Autodesk Fusion 360 part; units mm, degrees
(part 3 of 6)
sketch "Sketch23" plane through (0, 3, 0) normal (0, 1, 0) x (-1, 0, 0)
  line L0 (75.3451, 40.8932) -> (75.3451, 33.735)
  line L1 (75.3451, 33.735) -> (70.1693, 33.735)
  line L2 (70.1693, 33.735) -> (70.1693, 34.5798)
  line L3 (70.1693, 34.5798) -> (74.3978, 34.5798)
  line L4 (74.3978, 34.5798) -> (74.3978, 36.7721)
  line L5 (74.3978, 36.7721) -> (70.4379, 36.7721)
  line L6 (70.4379, 36.7721) -> (70.4379, 37.612)
  line L7 (70.4379, 37.612) -> (74.3978, 37.612)
  line L8 (74.3978, 37.612) -> (74.3978, 40.0485)
  line L9 (74.3978, 40.0485) -> (70.0033, 40.0485)
  line L10 (70.0033, 40.0485) -> (70.0033, 40.8932)
  line L11 (70.0033, 40.8932) -> (75.3451, 40.8932)
  line L12 (61.3265, 40.1071) -> (61.1996, 40.8835)
  spline S0 degree 3 poles (61.1996, 40.8835) (61.3164, 40.9062) (61.5358, 40.949) (61.7592, 40.9576) (61.8636, 40.9616) knots 0 0 0 0 0.035641 0.066952 0.066952 0.066952 0.066952
  spline S1 degree 3 poles (61.8636, 40.9616) (62.0074, 40.9588) (62.2648, 40.9539) (62.5014, 40.8542) (62.6058, 40.8102) knots 0 0 0 0 0.042649 0.076356 0.076356 0.076356 0.076356
  spline S2 degree 3 poles (62.6058, 40.8102) (62.6866, 40.7573) (62.8429, 40.6547) (62.9332, 40.4913) (62.9769, 40.4123) knots 0 0 0 0 0.028484 0.055146 0.055146 0.055146 0.055146
  spline S3 degree 3 poles (62.9769, 40.4123) (63.0078, 40.2852) (63.0904, 39.9452) (63.0867, 39.5944) (63.0843, 39.3747) knots 0 0 0 0 0.039108 0.104654 0.104654 0.104654 0.104654
  line L13 (63.0843, 39.3747) -> (63.0843, 36.3913)
  line L14 (63.0843, 36.3913) -> (63.7289, 36.3913)
  line L15 (63.7289, 36.3913) -> (63.7289, 35.7077)
  line L16 (63.7289, 35.7077) -> (63.0843, 35.7077)
  line L17 (63.0843, 35.7077) -> (63.0843, 34.4235)
  line L18 (63.0843, 34.4235) -> (62.2103, 33.8962)
  line L19 (62.2103, 33.8962) -> (62.2103, 35.7077)
  line L20 (62.2103, 35.7077) -> (61.3265, 35.7077)
  line L21 (61.3265, 35.7077) -> (61.3265, 36.3913)
  line L22 (61.3265, 36.3913) -> (62.2103, 36.3913)
  line L23 (62.2103, 36.3913) -> (62.2103, 39.4235)
  spline S4 degree 3 poles (62.2103, 39.4235) (62.2116, 39.5271) (62.2137, 39.6903) (62.1772, 39.8489) (62.1639, 39.9069) knots 0 0 0 0 0.030906 0.048705 0.048705 0.048705 0.048705
  spline S5 degree 3 poles (62.1639, 39.9069) (62.1458, 39.941) (62.1091, 40.0101) (62.045, 40.0551) (62.0126, 40.0778) knots 0 0 0 0 0.011413 0.023119 0.023119 0.023119 0.023119
  spline S6 degree 3 poles (62.0126, 40.0778) (61.9706, 40.0963) (61.8753, 40.1382) (61.7708, 40.1402) (61.7123, 40.1413) knots 0 0 0 0 0.013616 0.030961 0.030961 0.030961 0.030961
  spline S7 degree 3 poles (61.7123, 40.1413) (61.6556, 40.1393) (61.5265, 40.1347) (61.3984, 40.117) (61.3265, 40.1071) knots 0 0 0 0 0.016989 0.038747 0.038747 0.038747 0.038747
  line L24 (54.9154, 40.8932) -> (54.9154, 35.7077)
  line L25 (54.9154, 35.7077) -> (54.1244, 35.7077)
  line L26 (54.1244, 35.7077) -> (54.1244, 36.4938)
  spline S8 degree 3 poles (54.1244, 36.4938) (54.0363, 36.3341) (53.8864, 36.0624) (53.659, 35.8527) (53.5653, 35.7663) knots 0 0 0 0 0.05425 0.092273 0.092273 0.092273 0.092273
  spline S9 degree 3 poles (53.5653, 35.7663) (53.4779, 35.715) (53.3035, 35.6128) (53.1019, 35.5979) (53.0013, 35.5905) knots 0 0 0 0 0.029972 0.059777 0.059777 0.059777 0.059777
  spline S10 degree 3 poles (53.0013, 35.5905) (52.8491, 35.6045) (52.5282, 35.6341) (52.2462, 35.7912) (52.098, 35.8737) knots 0 0 0 0 0.045356 0.095599 0.095599 0.095599 0.095599
  line L27 (52.098, 35.8737) -> (52.4008, 36.6891)
  spline S11 degree 3 poles (52.4008, 36.6891) (52.5059, 36.6336) (52.7082, 36.5268) (52.9359, 36.5078) (53.0453, 36.4987) knots 0 0 0 0 0.03525 0.067826 0.067826 0.067826 0.067826
  spline S12 degree 3 poles (53.0453, 36.4987) (53.1389, 36.5059) (53.3259, 36.5203) (53.4839, 36.6215) (53.5629, 36.672) knots 0 0 0 0 0.027685 0.055345 0.055345 0.055345 0.055345
  spline S13 degree 3 poles (53.5629, 36.672) (53.6343, 36.7369) (53.7818, 36.8708) (53.8532, 37.057) (53.89, 37.153) knots 0 0 0 0 0.028537 0.058895 0.058895 0.058895 0.058895
  spline S14 degree 3 poles (53.89, 37.153) (53.9327, 37.3157) (54.021, 37.6518) (54.0312, 37.9992) (54.0365, 38.1784) knots 0 0 0 0 0.050287 0.103879 0.103879 0.103879 0.103879
  line L28 (54.0365, 38.1784) -> (54.0365, 40.8932)
  line L29 (54.0365, 40.8932) -> (54.9154, 40.8932)
  line L30 (31.9125, 39.2233) -> (31.0043, 39.3356)
  spline S15 degree 3 poles (31.0043, 39.3356) (31.0877, 39.5834) (31.2492, 40.0629) (31.6207, 40.4055) (31.8002, 40.571) knots 0 0 0 0 0.077034 0.149075 0.149075 0.149075 0.149075
  spline S16 degree 3 poles (31.8002, 40.571) (32.0151, 40.699) (32.4715, 40.9709) (33.0033, 40.9968) (33.2845, 41.0104) knots 0 0 0 0 0.073917 0.156923 0.156923 0.156923 0.156923
  spline S17 degree 3 poles (33.2845, 41.0104) (33.6385, 40.987) (34.3153, 40.9421) (34.8389, 40.514) (35.0887, 40.3097) knots 0 0 0 0 0.103483 0.197891 0.197891 0.197891 0.197891
  spline S18 degree 3 poles (35.0887, 40.3097) (35.2829, 40.039) (35.7022, 39.454) (35.7367, 38.7321) (35.7552, 38.3444) knots 0 0 0 0 0.097893 0.211487 0.211487 0.211487 0.211487
  spline S19 degree 3 poles (35.7552, 38.3444) (35.737, 37.9438) (35.703, 37.2003) (35.2776, 36.5932) (35.0814, 36.3132) knots 0 0 0 0 0.117426 0.217964 0.217964 0.217964 0.217964
  spline S20 degree 3 poles (35.0814, 36.3132) (34.8361, 36.1024) (34.3334, 35.6707) (33.6719, 35.6177) (33.3334, 35.5905) knots 0 0 0 0 0.094484 0.193557 0.193557 0.193557 0.193557
  spline S21 degree 3 poles (33.3334, 35.5905) (33.0049, 35.6175) (32.3613, 35.6704) (31.8732, 36.092) (31.6342, 36.2985) knots 0 0 0 0 0.096126 0.18838 0.18838 0.18838 0.18838
  spline S22 degree 3 poles (31.6342, 36.2985) (31.4422, 36.5731) (31.0258, 37.1688) (30.9928, 37.8977) (30.975, 38.2907) knots 0 0 0 0 0.098509 0.213708 0.213708 0.213708 0.213708
  spline S23 degree 3 poles (30.975, 38.2907) (30.9753, 38.3233) (30.976, 38.4014) (30.9784, 38.4795) (30.9799, 38.5251) knots 0 0 0 0 0.009766 0.023443 0.023443 0.023443 0.023443
  line L31 (30.9799, 38.5251) -> (34.847, 38.5251)
  spline S24 degree 3 poles (34.847, 38.5251) (34.8216, 38.7854) (34.7748, 39.2658) (34.4928, 39.6553) (34.3636, 39.8337) knots 0 0 0 0 0.076825 0.141746 0.141746 0.141746 0.141746
  spline S25 degree 3 poles (34.3636, 39.8337) (34.2089, 39.9661) (33.8964, 40.2335) (33.4865, 40.2696) (33.2797, 40.2878) knots 0 0 0 0 0.059532 0.120175 0.120175 0.120175 0.120175
  spline S26 degree 3 poles (33.2797, 40.2878) (33.1265, 40.2787) (32.8304, 40.2612) (32.5769, 40.1079) (32.4545, 40.0339) knots 0 0 0 0 0.045247 0.087501 0.087501 0.087501 0.087501
  spline S27 degree 3 poles (32.4545, 40.0339) (32.3441, 39.9297) (32.1023, 39.7015) (31.9793, 39.3917) (31.9125, 39.2233) knots 0 0 0 0 0.045001 0.098557 0.098557 0.098557 0.098557
  line L32 (39.3357, 58.6816) -> (39.3357, 47.9224)
  line L33 (39.3357, 47.9224) -> (38.1345, 47.9224)
  line L34 (38.1345, 47.9224) -> (38.1345, 48.9331)
  spline S28 degree 3 poles (38.1345, 48.9331) (37.9928, 48.7502) (37.7217, 48.4005) (37.3516, 48.1586) (37.1751, 48.0432) knots 0 0 0 0 0.068849 0.131677 0.131677 0.131677 0.131677
  spline S29 degree 3 poles (37.1751, 48.0432) (36.9808, 47.9568) (36.5687, 47.7734) (36.1173, 47.7558) (35.8787, 47.7466) knots 0 0 0 0 0.063189 0.134074 0.134074 0.134074 0.134074
  spline S30 degree 3 poles (35.8787, 47.7466) (35.5593, 47.766) (34.9341, 47.8041) (34.388, 48.1098) (34.1209, 48.2593) knots 0 0 0 0 0.094622 0.185218 0.185218 0.185218 0.185218
  spline S31 degree 3 poles (34.1209, 48.2593) (33.881, 48.4515) (33.3885, 48.8462) (33.1125, 49.4144) (32.971, 49.7058) knots 0 0 0 0 0.091026 0.186859 0.186859 0.186859 0.186859
  spline S32 degree 3 poles (32.971, 49.7058) (32.8578, 50.0289) (32.6256, 50.6916) (32.5973, 51.3934) (32.5828, 51.7529) knots 0 0 0 0 0.102108 0.20939 0.20939 0.20939 0.20939
  spline S33 degree 3 poles (32.5828, 51.7529) (32.5981, 52.1352) (32.6277, 52.8747) (32.8863, 53.5678) (33.0112, 53.9026) knots 0 0 0 0 0.113938 0.220434 0.220434 0.220434 0.220434
  spline S34 degree 3 poles (33.0112, 53.9026) (33.167, 54.2005) (33.4717, 54.7833) (33.9988, 55.1757) (34.2564, 55.3674) knots 0 0 0 0 0.099433 0.194467 0.194467 0.194467 0.194467
  spline S35 degree 3 poles (34.2564, 55.3674) (34.5294, 55.5159) (35.066, 55.8077) (35.6748, 55.8538) (35.9739, 55.8765) knots 0 0 0 0 0.09206 0.180958 0.180958 0.180958 0.180958
  spline S36 degree 3 poles (35.9739, 55.8765) (36.1854, 55.8662) (36.5971, 55.8462) (36.9737, 55.6793) (37.1567, 55.5981) knots 0 0 0 0 0.062916 0.122451 0.122451 0.122451 0.122451
  spline S37 degree 3 poles (37.1567, 55.5981) (37.3222, 55.501) (37.6455, 55.311) (37.8953, 55.0315) (38.0173, 54.895) knots 0 0 0 0 0.057158 0.111733 0.111733 0.111733 0.111733
  line L35 (38.0173, 54.895) -> (38.0173, 58.6816)
  line L36 (38.0173, 58.6816) -> (39.3357, 58.6816)
  line L37 (25.991, 46.4795) -> (25.991, 44.9634)
  line L38 (25.991, 44.9634) -> (24.6726, 44.9634)
  line L39 (24.6726, 44.9634) -> (24.6726, 46.4795)
  line L40 (24.6726, 46.4795) -> (25.991, 46.4795)
  line L41 (23.1931, 53.3789) -> (21.8894, 53.1738)
  spline S38 degree 3 poles (21.8894, 53.1738) (21.8413, 53.4156) (21.75, 53.8747) (21.4295, 54.2143) (21.2778, 54.375) knots 0 0 0 0 0.072267 0.137238 0.137238 0.137238 0.137238
  spline S39 degree 3 poles (21.2778, 54.375) (21.0827, 54.4965) (20.6552, 54.7628) (20.1499, 54.782) (19.8753, 54.7925) knots 0 0 0 0 0.067812 0.148597 0.148597 0.148597 0.148597
  spline S40 degree 3 poles (19.8753, 54.7925) (19.6043, 54.7862) (19.1216, 54.7751) (18.7087, 54.5301) (18.5276, 54.4226) knots 0 0 0 0 0.07964 0.141834 0.141834 0.141834 0.141834
  spline S41 degree 3 poles (18.5276, 54.4226) (18.3995, 54.2977) (18.1534, 54.0576) (18.1093, 53.7177) (18.0881, 53.5547) knots 0 0 0 0 0.051978 0.099855 0.099855 0.099855 0.099855
  spline S42 degree 3 poles (18.0881, 53.5547) (18.1051, 53.4132) (18.1394, 53.1267) (18.3631, 52.944) (18.4763, 52.8516) knots 0 0 0 0 0.04108 0.083169 0.083169 0.083169 0.083169
  spline S43 degree 3 poles (18.4763, 52.8516) (18.6325, 52.7814) (19.0657, 52.5869) (19.5282, 52.4758) (19.824, 52.4048) knots 0 0 0 0 0.051284 0.142232 0.142232 0.142232 0.142232
  spline S44 degree 3 poles (19.824, 52.4048) (20.2366, 52.3014) (20.9198, 52.1303) (21.575, 51.8731) (21.8345, 51.7712) knots 0 0 0 0 0.127433 0.210981 0.210981 0.210981 0.210981
  spline S45 degree 3 poles (21.8345, 51.7712) (22.0084, 51.6761) (22.346, 51.4914) (22.5737, 51.1817) (22.6841, 51.0315) knots 0 0 0 0 0.058662 0.113875 0.113875 0.113875 0.113875
  spline S46 degree 3 poles (22.6841, 51.0315) (22.7685, 50.8691) (22.9386, 50.5418) (22.9617, 50.1734) (22.9734, 49.9878) knots 0 0 0 0 0.054242 0.109375 0.109375 0.109375 0.109375
  spline S47 degree 3 poles (22.9734, 49.9878) (22.9638, 49.8183) (22.9449, 49.4823) (22.8048, 49.1763) (22.7354, 49.0247) knots 0 0 0 0 0.050432 0.099993 0.099993 0.099993 0.099993
  spline S48 degree 3 poles (22.7354, 49.0247) (22.6488, 48.8832) (22.4756, 48.6001) (22.2167, 48.3924) (22.0872, 48.2886) knots 0 0 0 0 0.049345 0.098743 0.098743 0.098743 0.098743
  spline S49 degree 3 poles (22.0872, 48.2886) (21.9683, 48.2138) (21.706, 48.0488) (21.4103, 47.9552) (21.2485, 47.904) knots 0 0 0 0 0.04196 0.092591 0.092591 0.092591 0.092591
  spline S50 degree 3 poles (21.2485, 47.904) (21.0661, 47.8581) (20.6922, 47.7641) (20.3069, 47.7525) (20.1096, 47.7466) knots 0 0 0 0 0.056276 0.115276 0.115276 0.115276 0.115276
  spline S51 degree 3 poles (20.1096, 47.7466) (19.8208, 47.755) (19.2727, 47.7709) (18.7494, 47.9334) (18.502, 48.0103) knots 0 0 0 0 0.08622 0.163589 0.163589 0.163589 0.163589
  spline S52 degree 3 poles (18.502, 48.0103) (18.2913, 48.0995) (17.8993, 48.2656) (17.6128, 48.5793) (17.4802, 48.7244) knots 0 0 0 0 0.067685 0.125961 0.125961 0.125961 0.125961
  spline S53 degree 3 poles (17.4802, 48.7244) (17.3776, 48.896) (17.1541, 49.2697) (17.0711, 49.6978) (17.0261, 49.9292) knots 0 0 0 0 0.059547 0.129628 0.129628 0.129628 0.129628
  line L42 (17.0261, 49.9292) -> (18.3152, 50.105)
  spline S54 degree 3 poles (18.3152, 50.105) (18.3559, 49.9178) (18.4349, 49.5552) (18.6973, 49.2939) (18.8242, 49.1675) knots 0 0 0 0 0.056141 0.108715 0.108715 0.108715 0.108715
  spline S55 degree 3 poles (18.8242, 49.1675) (18.9894, 49.0694) (19.3548, 48.8527) (19.781, 48.8384) (20.0144, 48.8306) knots 0 0 0 0 0.056748 0.125473 0.125473 0.125473 0.125473
  spline S56 degree 3 poles (20.0144, 48.8306) (20.2797, 48.8327) (20.7368, 48.8364) (21.1412, 49.0438) (21.3108, 49.1309) knots 0 0 0 0 0.078181 0.134683 0.134683 0.134683 0.134683
  spline S57 degree 3 poles (21.3108, 49.1309) (21.4239, 49.2309) (21.6378, 49.4202) (21.6794, 49.7014) (21.699, 49.834) knots 0 0 0 0 0.043702 0.082651 0.082651 0.082651 0.082651
  spline S58 degree 3 poles (21.699, 49.834) (21.6921, 49.9175) (21.6784, 50.0852) (21.5848, 50.2251) (21.5379, 50.2954) knots 0 0 0 0 0.024684 0.0496 0.0496 0.0496 0.0496
  spline S59 degree 3 poles (21.5379, 50.2954) (21.4722, 50.3648) (21.3286, 50.5167) (21.1367, 50.6011) (21.0325, 50.647) knots 0 0 0 0 0.02837 0.062115 0.062115 0.062115 0.062115
  spline S60 degree 3 poles (21.0325, 50.647) (20.9027, 50.6879) (20.5172, 50.8093) (20.1268, 50.9143) (19.8679, 50.9839) knots 0 0 0 0 0.040831 0.121242 0.121242 0.121242 0.121242
  spline S61 degree 3 poles (19.8679, 50.9839) (19.4697, 51.0896) (18.8099, 51.2649) (18.1698, 51.5016) (17.916, 51.5955) knots 0 0 0 0 0.123506 0.204645 0.204645 0.204645 0.204645
  spline S62 degree 3 poles (17.916, 51.5955) (17.7429, 51.682) (17.4043, 51.8513) (17.165, 52.1444) (17.0481, 52.2876) knots 0 0 0 0 0.057342 0.11214 0.11214 0.11214 0.11214
  spline S63 degree 3 poles (17.0481, 52.2876) (16.9563, 52.4535) (16.7625, 52.8039) (16.7433, 53.2046) (16.7332, 53.4155) knots 0 0 0 0 0.056117 0.118505 0.118505 0.118505 0.118505
  spline S64 degree 3 poles (16.7332, 53.4155) (16.7501, 53.6335) (16.7846, 54.0761) (17.0055, 54.4614) (17.1177, 54.657) knots 0 0 0 0 0.064713 0.13142 0.13142 0.13142 0.13142
  spline S65 degree 3 poles (17.1177, 54.657) (17.2639, 54.8417) (17.5664, 55.2241) (18.0021, 55.4441) (18.2273, 55.5579) knots 0 0 0 0 0.0698 0.14446 0.14446 0.14446 0.14446
  spline S66 degree 3 poles (18.2273, 55.5579) (18.4822, 55.6507) (19.0119, 55.8437) (19.5756, 55.8653) (19.8679, 55.8765) knots 0 0 0 0 0.080881 0.168038 0.168038 0.168038 0.168038
  spline S67 degree 3 poles (19.8679, 55.8765) (20.3248, 55.8636) (21.1496, 55.8403) (21.8612, 55.4297) (22.1787, 55.2466) knots 0 0 0 0 0.1345 0.242846 0.242846 0.242846 0.242846
  spline S68 degree 3 poles (22.1787, 55.2466) (22.4214, 55.0003) (22.9373, 54.4768) (23.1046, 53.759) (23.1931, 53.3789) knots 0 0 0 0 0.101736 0.21624 0.21624 0.21624 0.21624
  line L43 (25.991, 55.7007) -> (25.991, 47.9224)
  line L44 (25.991, 47.9224) -> (24.6726, 47.9224)
  line L45 (24.6726, 47.9224) -> (24.6726, 55.7007)
  line L46 (24.6726, 55.7007) -> (25.991, 55.7007)
  line L47 (31.0081, 55.7007) -> (31.0081, 47.9224)
  line L48 (31.0081, 47.9224) -> (29.8215, 47.9224)
  line L49 (29.8215, 47.9224) -> (29.8215, 49.1016)
  spline S69 degree 3 poles (29.8215, 49.1016) (29.6894, 48.862) (29.4646, 48.4545) (29.1235, 48.1399) (28.9829, 48.0103) knots 0 0 0 0 0.081375 0.138409 0.138409 0.138409 0.138409
  spline S70 degree 3 poles (28.9829, 48.0103) (28.8518, 47.9333) (28.5902, 47.78) (28.2878, 47.7577) (28.137, 47.7466) knots 0 0 0 0 0.044958 0.089666 0.089666 0.089666 0.089666
  spline S71 degree 3 poles (28.137, 47.7466) (27.9086, 47.7676) (27.4272, 47.812) (27.0043, 48.0476) (26.782, 48.1714) knots 0 0 0 0 0.068034 0.143398 0.143398 0.143398 0.143398
  line L50 (26.782, 48.1714) -> (27.2361, 49.3945)
  spline S72 degree 3 poles (27.2361, 49.3945) (27.3938, 49.3113) (27.6972, 49.151) (28.0388, 49.1226) (28.2029, 49.1089) knots 0 0 0 0 0.052874 0.101739 0.101739 0.101739 0.101739
  spline S73 degree 3 poles (28.2029, 49.1089) (28.3432, 49.1197) (28.6238, 49.1413) (28.8608, 49.2931) (28.9793, 49.3689) knots 0 0 0 0 0.041528 0.083017 0.083017 0.083017 0.083017
  spline S74 degree 3 poles (28.9793, 49.3689) (29.0865, 49.4662) (29.3077, 49.667) (29.4148, 49.9464) (29.47, 50.0903) knots 0 0 0 0 0.042806 0.088343 0.088343 0.088343 0.088343
  spline S75 degree 3 poles (29.47, 50.0903) (29.534, 50.3344) (29.6664, 50.8385) (29.6818, 51.3596) (29.6897, 51.6284) knots 0 0 0 0 0.075431 0.155819 0.155819 0.155819 0.155819
  line L51 (29.6897, 51.6284) -> (29.6897, 55.7007)
  line L52 (29.6897, 55.7007) -> (31.0081, 55.7007)
  line L53 (47.3484, 53.1958) -> (45.9861, 53.3643)
  spline S76 degree 3 poles (45.9861, 53.3643) (46.1113, 53.7359) (46.3535, 54.4552) (46.9107, 54.969) (47.1799, 55.2173) knots 0 0 0 0 0.115551 0.223613 0.223613 0.223613 0.223613
  spline S77 degree 3 poles (47.1799, 55.2173) (47.5024, 55.4094) (48.1869, 55.8172) (48.9846, 55.8559) (49.4065, 55.8765) knots 0 0 0 0 0.110875 0.235384 0.235384 0.235384 0.235384
  spline S78 degree 3 poles (49.4065, 55.8765) (49.9374, 55.8413) (50.9526, 55.774) (51.7381, 55.1318) (52.1128, 54.8254) knots 0 0 0 0 0.155225 0.296837 0.296837 0.296837 0.296837
  spline S79 degree 3 poles (52.1128, 54.8254) (52.404, 54.4193) (53.033, 53.5417) (53.0848, 52.459) (53.1126, 51.8774) knots 0 0 0 0 0.146839 0.31723 0.31723 0.31723 0.31723
  spline S80 degree 3 poles (53.1126, 51.8774) (53.0851, 51.2766) (53.0342, 50.1613) (52.3961, 49.2506) (52.1018, 48.8306) knots 0 0 0 0 0.176138 0.326947 0.326947 0.326947 0.326947
  spline S81 degree 3 poles (52.1018, 48.8306) (51.7338, 48.5145) (50.9798, 47.8669) (49.9876, 47.7873) (49.4797, 47.7466) knots 0 0 0 0 0.141726 0.290335 0.290335 0.290335 0.290335
  spline S82 degree 3 poles (49.4797, 47.7466) (48.9871, 47.7871) (48.0216, 47.8664) (47.2895, 48.4989) (46.9309, 48.8086) knots 0 0 0 0 0.144189 0.28257 0.28257 0.28257 0.28257
  spline S83 degree 3 poles (46.9309, 48.8086) (46.643, 49.2205) (46.0184, 50.114) (45.9688, 51.2074) (45.9421, 51.7969) knots 0 0 0 0 0.147764 0.320562 0.320562 0.320562 0.320562
  spline S84 degree 3 poles (45.9421, 51.7969) (45.9426, 51.8457) (45.9437, 51.9629) (45.9474, 52.0801) (45.9495, 52.1484) knots 0 0 0 0 0.01465 0.035165 0.035165 0.035165 0.035165
  line L54 (45.9495, 52.1484) -> (51.7503, 52.1484)
  spline S85 degree 3 poles (51.7503, 52.1484) (51.7122, 52.539) (51.6419, 53.2596) (51.2189, 53.8438) (51.0252, 54.1113) knots 0 0 0 0 0.115238 0.212619 0.212619 0.212619 0.212619
  spline S86 degree 3 poles (51.0252, 54.1113) (50.793, 54.31) (50.3243, 54.711) (49.7094, 54.7652) (49.3992, 54.7925) knots 0 0 0 0 0.089299 0.180262 0.180262 0.180262 0.180262
  spline S87 degree 3 poles (49.3992, 54.7925) (49.1695, 54.7789) (48.7253, 54.7526) (48.345, 54.5227) (48.1614, 54.4116) knots 0 0 0 0 0.067871 0.131252 0.131252 0.131252 0.131252
  spline S88 degree 3 poles (48.1614, 54.4116) (47.9958, 54.2553) (47.6332, 53.913) (47.4487, 53.4483) (47.3484, 53.1958) knots 0 0 0 0 0.067501 0.147835 0.147835 0.147835 0.147835
  line L55 (65.1829, 55.7007) -> (65.1829, 47.9224)
  line L56 (65.1829, 47.9224) -> (63.9963, 47.9224)
  line L57 (63.9963, 47.9224) -> (63.9963, 49.0283)
  spline S89 degree 3 poles (63.9963, 49.0283) (63.6751, 48.6545) (63.0232, 47.8958) (62.0264, 47.7968) (61.5208, 47.7466) knots 0 0 0 0 0.142165 0.288537 0.288537 0.288537 0.288537
  spline S90 degree 3 poles (61.5208, 47.7466) (61.2936, 47.7561) (60.8496, 47.7746) (60.4319, 47.9256) (60.228, 47.9993) knots 0 0 0 0 0.067769 0.132408 0.132408 0.132408 0.132408
  spline S91 degree 3 poles (60.228, 47.9993) (60.0475, 48.0852) (59.7079, 48.2468) (59.4611, 48.5296) (59.3455, 48.6621) knots 0 0 0 0 0.059243 0.111422 0.111422 0.111422 0.111422
  spline S92 degree 3 poles (59.3455, 48.6621) (59.2545, 48.8083) (59.0662, 49.111) (58.9799, 49.4572) (58.9353, 49.6362) knots 0 0 0 0 0.051309 0.106275 0.106275 0.106275 0.106275
  spline S93 degree 3 poles (58.9353, 49.6362) (58.9142, 49.8039) (58.8606, 50.2292) (58.8615, 50.6581) (58.8621, 50.918) knots 0 0 0 0 0.050653 0.128494 0.128494 0.128494 0.128494
  line L58 (58.8621, 50.918) -> (58.8621, 55.7007)
  line L59 (58.8621, 55.7007) -> (60.1804, 55.7007)
  line L60 (60.1804, 55.7007) -> (60.1804, 50.9692)
  spline S94 degree 3 poles (60.1804, 50.9692) (60.1817, 50.7329) (60.1839, 50.3244) (60.2896, 49.9305) (60.3342, 49.7644) knots 0 0 0 0 0.070509 0.1219 0.1219 0.1219 0.1219
  spline S95 degree 3 poles (60.3342, 49.7644) (60.3966, 49.6373) (60.5238, 49.3784) (60.7597, 49.212) (60.8799, 49.1272) knots 0 0 0 0 0.04175 0.085098 0.085098 0.085098 0.085098
  spline S96 degree 3 poles (60.8799, 49.1272) (61.0192, 49.0578) (61.3084, 48.9137) (61.6316, 48.8975) (61.7991, 48.8892) knots 0 0 0 0 0.046164 0.095868 0.095868 0.095868 0.095868
  spline S97 degree 3 poles (61.7991, 48.8892) (62.0692, 48.9105) (62.6041, 48.9529) (63.0381, 49.2679) (63.2529, 49.4238) knots 0 0 0 0 0.079591 0.15761 0.15761 0.15761 0.15761
  spline S98 degree 3 poles (63.2529, 49.4238) (63.4301, 49.6738) (63.8559, 50.2745) (63.8613, 51.0183) (63.8645, 51.4526) knots 0 0 0 0 0.090016 0.216372 0.216372 0.216372 0.216372
  line L61 (63.8645, 51.4526) -> (63.8645, 55.7007)
  line L62 (63.8645, 55.7007) -> (65.1829, 55.7007)
  line L63 (77.2473, 74.5713) -> (77.2473, 60.2549)
  line L64 (77.2473, 60.2549) -> (66.8957, 60.2549)
  line L65 (66.8957, 60.2549) -> (66.8957, 61.9443)
  line L66 (66.8957, 61.9443) -> (75.3528, 61.9443)
  line L67 (75.3528, 61.9443) -> (75.3528, 66.3291)
  line L68 (75.3528, 66.3291) -> (67.4328, 66.3291)
  line L69 (67.4328, 66.3291) -> (67.4328, 68.0088)
  line L70 (67.4328, 68.0088) -> (75.3528, 68.0088)
  line L71 (75.3528, 68.0088) -> (75.3528, 72.8818)
  line L72 (75.3528, 72.8818) -> (66.5637, 72.8818)
  line L73 (66.5637, 72.8818) -> (66.5637, 74.5713)
  line L74 (66.5637, 74.5713) -> (77.2473, 74.5713)
  line L75 (49.2102, 72.999) -> (48.9563, 74.5517)
  spline S99 degree 3 poles (48.9563, 74.5517) (49.1899, 74.5972) (49.6288, 74.6827) (50.0755, 74.6999) (50.2844, 74.708) knots 0 0 0 0 0.071282 0.133904 0.133904 0.133904 0.133904
  spline S100 degree 3 poles (50.2844, 74.708) (50.5719, 74.7024) (51.0867, 74.6925) (51.5599, 74.4932) (51.7688, 74.4052) knots 0 0 0 0 0.085297 0.152712 0.152712 0.152712 0.152712
  spline S101 degree 3 poles (51.7688, 74.4052) (51.9303, 74.2993) (52.2429, 74.0941) (52.4236, 73.7673) (52.511, 73.6093) knots 0 0 0 0 0.056968 0.110293 0.110293 0.110293 0.110293
  spline S102 degree 3 poles (52.511, 73.6093) (52.5727, 73.3552) (52.738, 72.6752) (52.7305, 71.9736) (52.7258, 71.5341) knots 0 0 0 0 0.078216 0.209307 0.209307 0.209307 0.209307
  line L76 (52.7258, 71.5341) -> (52.7258, 65.5674)
  line L77 (52.7258, 65.5674) -> (54.0149, 65.5674)
  line L78 (54.0149, 65.5674) -> (54.0149, 64.2002)
  line L79 (54.0149, 64.2002) -> (52.7258, 64.2002)
  line L80 (52.7258, 64.2002) -> (52.7258, 61.6318)
  line L81 (52.7258, 61.6318) -> (50.9778, 60.5771)
  line L82 (50.9778, 60.5771) -> (50.9778, 64.2002)
  line L83 (50.9778, 64.2002) -> (49.2102, 64.2002)
  line L84 (49.2102, 64.2002) -> (49.2102, 65.5674)
  line L85 (49.2102, 65.5674) -> (50.9778, 65.5674)
  line L86 (50.9778, 65.5674) -> (50.9778, 71.6318)
  spline S103 degree 3 poles (50.9778, 71.6318) (50.9804, 71.8389) (50.9844, 72.1653) (50.9116, 72.4826) (50.885, 72.5986) knots 0 0 0 0 0.061811 0.09741 0.09741 0.09741 0.09741
  spline S104 degree 3 poles (50.885, 72.5986) (50.8488, 72.6668) (50.7753, 72.805) (50.6472, 72.8949) (50.5823, 72.9404) knots 0 0 0 0 0.022826 0.046239 0.046239 0.046239 0.046239
  spline S105 degree 3 poles (50.5823, 72.9404) (50.4984, 72.9773) (50.3077, 73.0612) (50.0987, 73.0651) (49.9817, 73.0674) knots 0 0 0 0 0.027232 0.061923 0.061923 0.061923 0.061923
  spline S106 degree 3 poles (49.9817, 73.0674) (49.8684, 73.0633) (49.6101, 73.0542) (49.354, 73.0188) (49.2102, 72.999) knots 0 0 0 0 0.033979 0.077495 0.077495 0.077495 0.077495
  line L87 (36.3879, 74.5713) -> (36.3879, 64.2002)
  line L88 (36.3879, 64.2002) -> (34.8059, 64.2002)
  line L89 (34.8059, 64.2002) -> (34.8059, 65.7724)
  spline S107 degree 3 poles (34.8059, 65.7724) (34.6297, 65.453) (34.3299, 64.9096) (33.8751, 64.4902) (33.6877, 64.3174) knots 0 0 0 0 0.1085 0.184546 0.184546 0.184546 0.184546
  spline S108 degree 3 poles (33.6877, 64.3174) (33.5128, 64.2148) (33.164, 64.0103) (32.7608, 63.9806) (32.5598, 63.9658) knots 0 0 0 0 0.059943 0.119555 0.119555 0.119555 0.119555
  spline S109 degree 3 poles (32.5598, 63.9658) (32.2553, 63.9939) (31.6135, 64.053) (31.0495, 64.3671) (30.7532, 64.5322) knots 0 0 0 0 0.090712 0.191197 0.191197 0.191197 0.191197
  line L90 (30.7532, 64.5322) -> (31.3586, 66.1631)
  spline S110 degree 3 poles (31.3586, 66.1631) (31.5689, 66.052) (31.9735, 65.8384) (32.4289, 65.8004) (32.6477, 65.7822) knots 0 0 0 0 0.070499 0.135652 0.135652 0.135652 0.135652
  spline S111 degree 3 poles (32.6477, 65.7822) (32.8348, 65.7966) (33.2089, 65.8254) (33.5249, 66.0278) (33.6828, 66.1289) knots 0 0 0 0 0.05537 0.110689 0.110689 0.110689 0.110689
  spline S112 degree 3 poles (33.6828, 66.1289) (33.8258, 66.2586) (34.1208, 66.5264) (34.2635, 66.8988) (34.3371, 67.0908) knots 0 0 0 0 0.057074 0.117791 0.117791 0.117791 0.117791
  spline S113 degree 3 poles (34.3371, 67.0908) (34.4226, 67.4162) (34.599, 68.0883) (34.6195, 68.7831) (34.6301, 69.1416) knots 0 0 0 0 0.100574 0.207758 0.207758 0.207758 0.207758
  line L91 (34.6301, 69.1416) -> (34.6301, 74.5713)
  line L92 (34.6301, 74.5713) -> (36.3879, 74.5713)
  line L93 (-9.6179, 71.2314) -> (-11.4343, 71.456)
  spline S114 degree 3 poles (-11.4343, 71.456) (-11.2675, 71.9516) (-10.9445, 72.9106) (-10.2016, 73.5957) (-9.8425, 73.9267) knots 0 0 0 0 0.154068 0.298151 0.298151 0.298151 0.298151
  spline S115 degree 3 poles (-9.8425, 73.9267) (-9.4126, 74.1828) (-8.4999, 74.7266) (-7.4364, 74.7783) (-6.8738, 74.8056) knots 0 0 0 0 0.147834 0.313845 0.313845 0.313845 0.313845
  spline S116 degree 3 poles (-6.8738, 74.8056) (-6.1659, 74.7587) (-4.8123, 74.669) (-3.765, 73.8128) (-3.2654, 73.4043) knots 0 0 0 0 0.206966 0.395783 0.395783 0.395783 0.395783
  spline S117 degree 3 poles (-3.2654, 73.4043) (-2.8772, 72.8627) (-2.0385, 71.6927) (-1.9695, 70.249) (-1.9324, 69.4736) knots 0 0 0 0 0.195785 0.422974 0.422974 0.422974 0.422974
  spline S118 degree 3 poles (-1.9324, 69.4736) (-1.9689, 68.6725) (-2.0368, 67.1854) (-2.8876, 65.9712) (-3.28, 65.4111) knots 0 0 0 0 0.234851 0.435929 0.435929 0.435929 0.435929
  spline S119 degree 3 poles (-3.28, 65.4111) (-3.7708, 64.9896) (-4.776, 64.1262) (-6.099, 64.0201) (-6.7761, 63.9658) knots 0 0 0 0 0.188967 0.387114 0.387114 0.387114 0.387114
  spline S120 degree 3 poles (-6.7761, 63.9658) (-7.433, 64.0198) (-8.7203, 64.1256) (-9.6965, 64.9688) (-10.1746, 65.3818) knots 0 0 0 0 0.192252 0.37676 0.37676 0.37676 0.37676
  spline S121 degree 3 poles (-10.1746, 65.3818) (-10.5585, 65.931) (-11.3913, 67.1223) (-11.4573, 68.5803) (-11.4929, 69.3662) knots 0 0 0 0 0.197018 0.427415 0.427415 0.427415 0.427415
  spline S122 degree 3 poles (-11.4929, 69.3662) (-11.4923, 69.4313) (-11.4908, 69.5876) (-11.486, 69.7438) (-11.4832, 69.8349) knots 0 0 0 0 0.019533 0.046886 0.046886 0.046886 0.046886
  line L94 (-11.4832, 69.8349) -> (-3.7488, 69.8349)
  spline S123 degree 3 poles (-3.7488, 69.8349) (-3.7996, 70.3557) (-3.8933, 71.3165) (-4.4573, 72.0954) (-4.7156, 72.4521) knots 0 0 0 0 0.153651 0.283492 0.283492 0.283492 0.283492
  spline S124 degree 3 poles (-4.7156, 72.4521) (-5.0252, 72.717) (-5.6501, 73.2517) (-6.4699, 73.3239) (-6.8836, 73.3603) knots 0 0 0 0 0.119065 0.24035 0.24035 0.24035 0.24035
  spline S125 degree 3 poles (-6.8836, 73.3603) (-7.1898, 73.3422) (-7.7821, 73.3072) (-8.2891, 73.0006) (-8.534, 72.8525) knots 0 0 0 0 0.090495 0.175003 0.175003 0.175003 0.175003
  spline S126 degree 3 poles (-8.534, 72.8525) (-8.7547, 72.6441) (-9.2382, 72.1877) (-9.4842, 71.5681) (-9.6179, 71.2314) knots 0 0 0 0 0.090002 0.197114 0.197114 0.197114 0.197114
  line L95 (80, 80) -> (-25, 80)
  line L96 (-25, 80) -> (-25, 30)
  line L97 (-25, 30) -> (80, 30)
  line L98 (80, 30) -> (80, 80)
  line L99 (64.1711, 74.5713) -> (64.1711, 64.2002)
  line L100 (64.1711, 64.2002) -> (62.5891, 64.2002)
  line L101 (62.5891, 64.2002) -> (62.5891, 65.6748)
  spline S127 degree 3 poles (62.5891, 65.6748) (62.1608, 65.1763) (61.2915, 64.1647) (59.9625, 64.0328) (59.2883, 63.9658) knots 0 0 0 0 0.189553 0.384716 0.384716 0.384716 0.384716
  spline S128 degree 3 poles (59.2883, 63.9658) (58.9854, 63.9785) (58.3935, 64.0032) (57.8366, 64.2045) (57.5647, 64.3027) knots 0 0 0 0 0.090359 0.176544 0.176544 0.176544 0.176544
  spline S129 degree 3 poles (57.5647, 64.3027) (57.3239, 64.4173) (56.8712, 64.6327) (56.5421, 65.0099) (56.3879, 65.1865) knots 0 0 0 0 0.078991 0.148563 0.148563 0.148563 0.148563
  spline S130 degree 3 poles (56.3879, 65.1865) (56.2667, 65.3814) (56.0155, 65.785) (55.9005, 66.2466) (55.841, 66.4853) knots 0 0 0 0 0.068412 0.1417 0.1417 0.1417 0.1417
  spline S131 degree 3 poles (55.841, 66.4853) (55.8129, 66.7089) (55.7414, 67.276) (55.7426, 67.8478) (55.7434, 68.1943) knots 0 0 0 0 0.067537 0.171325 0.171325 0.171325 0.171325
  line L102 (55.7434, 68.1943) -> (55.7434, 74.5713)
  line L103 (55.7434, 74.5713) -> (57.5012, 74.5713)
  line L104 (57.5012, 74.5713) -> (57.5012, 68.2627)
  spline S132 degree 3 poles (57.5012, 68.2627) (57.5029, 67.9476) (57.5058, 67.4028) (57.6468, 66.8776) (57.7063, 66.6562) knots 0 0 0 0 0.094012 0.162533 0.162533 0.162533 0.162533
  spline S133 degree 3 poles (57.7063, 66.6562) (57.7895, 66.4868) (57.959, 66.1415) (58.2736, 65.9196) (58.4338, 65.8066) knots 0 0 0 0 0.055666 0.113464 0.113464 0.113464 0.113464
  spline S134 degree 3 poles (58.4338, 65.8066) (58.6195, 65.7141) (59.0052, 65.5219) (59.436, 65.5004) (59.6594, 65.4892) knots 0 0 0 0 0.061552 0.127824 0.127824 0.127824 0.127824
  spline S135 degree 3 poles (59.6594, 65.4892) (60.0196, 65.5177) (60.7327, 65.5742) (61.3114, 65.9942) (61.5979, 66.2021) knots 0 0 0 0 0.106122 0.210147 0.210147 0.210147 0.210147
  spline S136 degree 3 poles (61.5979, 66.2021) (61.8341, 66.5354) (62.4018, 67.3364) (62.4091, 68.3281) (62.4133, 68.9072) knots 0 0 0 0 0.120022 0.288496 0.288496 0.288496 0.288496
  line L105 (62.4133, 68.9072) -> (62.4133, 74.5713)
  line L106 (62.4133, 74.5713) -> (64.1711, 74.5713)
  line L107 (40.3918, 71.2314) -> (38.5754, 71.456)
  spline S137 degree 3 poles (38.5754, 71.456) (38.7423, 71.9516) (39.0652, 72.9106) (39.8082, 73.5957) (40.1672, 73.9267) knots 0 0 0 0 0.154068 0.298151 0.298151 0.298151 0.298151
  spline S138 degree 3 poles (40.1672, 73.9267) (40.5971, 74.1828) (41.5099, 74.7266) (42.5734, 74.7783) (43.136, 74.8056) knots 0 0 0 0 0.147834 0.313845 0.313845 0.313845 0.313845
  spline S139 degree 3 poles (43.136, 74.8056) (43.8438, 74.7587) (45.1975, 74.669) (46.2447, 73.8128) (46.7444, 73.4043) knots 0 0 0 0 0.206966 0.395783 0.395783 0.395783 0.395783
  spline S140 degree 3 poles (46.7444, 73.4043) (47.1326, 72.8627) (47.9713, 71.6927) (48.0403, 70.249) (48.0774, 69.4736) knots 0 0 0 0 0.195785 0.422974 0.422974 0.422974 0.422974
  spline S141 degree 3 poles (48.0774, 69.4736) (48.0408, 68.6725) (47.973, 67.1854) (47.1222, 65.9712) (46.7297, 65.4111) knots 0 0 0 0 0.234851 0.435929 0.435929 0.435929 0.435929
  spline S142 degree 3 poles (46.7297, 65.4111) (46.239, 64.9896) (45.2337, 64.1262) (43.9108, 64.0201) (43.2336, 63.9658) knots 0 0 0 0 0.188967 0.387114 0.387114 0.387114 0.387114
  spline S143 degree 3 poles (43.2336, 63.9658) (42.5767, 64.0198) (41.2894, 64.1256) (40.3132, 64.9688) (39.8352, 65.3818) knots 0 0 0 0 0.192252 0.37676 0.37676 0.37676 0.37676
  spline S144 degree 3 poles (39.8352, 65.3818) (39.4513, 65.931) (38.6184, 67.1223) (38.5524, 68.5803) (38.5168, 69.3662) knots 0 0 0 0 0.197018 0.427415 0.427415 0.427415 0.427415
  spline S145 degree 3 poles (38.5168, 69.3662) (38.5175, 69.4313) (38.5189, 69.5876) (38.5238, 69.7438) (38.5266, 69.8349) knots 0 0 0 0 0.019533 0.046886 0.046886 0.046886 0.046886
  line L108 (38.5266, 69.8349) -> (46.261, 69.8349)
  spline S146 degree 3 poles (46.261, 69.8349) (46.2102, 70.3557) (46.1165, 71.3165) (45.5525, 72.0954) (45.2942, 72.4521) knots 0 0 0 0 0.153651 0.283492 0.283492 0.283492 0.283492
  spline S147 degree 3 poles (45.2942, 72.4521) (44.9846, 72.717) (44.3597, 73.2517) (43.5399, 73.3239) (43.1262, 73.3603) knots 0 0 0 0 0.119065 0.24035 0.24035 0.24035 0.24035
  spline S148 degree 3 poles (43.1262, 73.3603) (42.8199, 73.3422) (42.2277, 73.3072) (41.7207, 73.0006) (41.4758, 72.8525) knots 0 0 0 0 0.090495 0.175003 0.175003 0.175003 0.175003
  spline S149 degree 3 poles (41.4758, 72.8525) (41.255, 72.6441) (40.7715, 72.1877) (40.5255, 71.5681) (40.3918, 71.2314) knots 0 0 0 0 0.090002 0.197114 0.197114 0.197114 0.197114
  line L109 (18.6047, 74.5713) -> (18.6047, 64.2002)
  line L110 (18.6047, 64.2002) -> (17.0227, 64.2002)
  line L111 (17.0227, 64.2002) -> (17.0227, 65.7724)
  spline S150 degree 3 poles (17.0227, 65.7724) (16.8465, 65.453) (16.5467, 64.9096) (16.0919, 64.4902) (15.9045, 64.3174) knots 0 0 0 0 0.1085 0.184546 0.184546 0.184546 0.184546
  spline S151 degree 3 poles (15.9045, 64.3174) (15.7296, 64.2148) (15.3808, 64.0103) (14.9776, 63.9806) (14.7766, 63.9658) knots 0 0 0 0 0.059943 0.119555 0.119555 0.119555 0.119555
  spline S152 degree 3 poles (14.7766, 63.9658) (14.4721, 63.9939) (13.8303, 64.053) (13.2663, 64.3671) (12.97, 64.5322) knots 0 0 0 0 0.090712 0.191197 0.191197 0.191197 0.191197
  line L112 (12.97, 64.5322) -> (13.5754, 66.1631)
  spline S153 degree 3 poles (13.5754, 66.1631) (13.7857, 66.052) (14.1903, 65.8384) (14.6457, 65.8004) (14.8645, 65.7822) knots 0 0 0 0 0.070499 0.135652 0.135652 0.135652 0.135652
  spline S154 degree 3 poles (14.8645, 65.7822) (15.0516, 65.7966) (15.4257, 65.8254) (15.7417, 66.0278) (15.8996, 66.1289) knots 0 0 0 0 0.05537 0.110689 0.110689 0.110689 0.110689
  spline S155 degree 3 poles (15.8996, 66.1289) (16.0426, 66.2586) (16.3376, 66.5264) (16.4803, 66.8988) (16.5539, 67.0908) knots 0 0 0 0 0.057074 0.117791 0.117791 0.117791 0.117791
  spline S156 degree 3 poles (16.5539, 67.0908) (16.6394, 67.4162) (16.8158, 68.0883) (16.8363, 68.7831) (16.8469, 69.1416) knots 0 0 0 0 0.100574 0.207758 0.207758 0.207758 0.207758
  line L113 (16.8469, 69.1416) -> (16.8469, 74.5713)
  line L114 (16.8469, 74.5713) -> (18.6047, 74.5713)
  line L115 (11.9153, 74.5713) -> (11.9153, 64.2002)
  line L116 (11.9153, 64.2002) -> (10.1575, 64.2002)
  line L117 (10.1575, 64.2002) -> (10.1575, 74.5713)
  line L118 (10.1575, 74.5713) -> (11.9153, 74.5713)
  line L119 (8.1848, 71.4756) -> (6.4465, 71.2021)
  spline S157 degree 3 poles (6.4465, 71.2021) (6.3824, 71.5245) (6.2606, 72.1366) (5.8334, 72.5894) (5.6311, 72.8037) knots 0 0 0 0 0.096356 0.182984 0.182984 0.182984 0.182984
  spline S158 degree 3 poles (5.6311, 72.8037) (5.3709, 72.9657) (4.8009, 73.3208) (4.1272, 73.3464) (3.761, 73.3603) knots 0 0 0 0 0.090416 0.19813 0.19813 0.19813 0.19813
  spline S159 degree 3 poles (3.761, 73.3603) (3.3996, 73.352) (2.7562, 73.3372) (2.2055, 73.0104) (1.9641, 72.8672) knots 0 0 0 0 0.106187 0.189111 0.189111 0.189111 0.189111
  spline S160 degree 3 poles (1.9641, 72.8672) (1.7933, 72.7006) (1.4651, 72.3805) (1.4063, 71.9272) (1.3782, 71.7099) knots 0 0 0 0 0.069303 0.133141 0.133141 0.133141 0.133141
  spline S161 degree 3 poles (1.3782, 71.7099) (1.4008, 71.5213) (1.4465, 71.1393) (1.7448, 70.8957) (1.8957, 70.7724) knots 0 0 0 0 0.054773 0.110892 0.110892 0.110892 0.110892
  spline S162 degree 3 poles (1.8957, 70.7724) (2.104, 70.6789) (2.6816, 70.4195) (3.2983, 70.2714) (3.6926, 70.1767) knots 0 0 0 0 0.068379 0.189643 0.189643 0.189643 0.189643
  spline S163 degree 3 poles (3.6926, 70.1767) (4.2428, 70.0389) (5.1537, 69.8107) (6.0273, 69.4678) (6.3733, 69.332) knots 0 0 0 0 0.169911 0.281309 0.281309 0.281309 0.281309
  spline S164 degree 3 poles (6.3733, 69.332) (6.6051, 69.2051) (7.0553, 68.9589) (7.3589, 68.5459) (7.5061, 68.3457) knots 0 0 0 0 0.078215 0.151833 0.151833 0.151833 0.151833
  spline S165 degree 3 poles (7.5061, 68.3457) (7.6186, 68.1292) (7.8455, 67.6927) (7.8763, 67.2016) (7.8918, 66.9541) knots 0 0 0 0 0.072323 0.145834 0.145834 0.145834 0.145834
  spline S166 degree 3 poles (7.8918, 66.9541) (7.8791, 66.7281) (7.8538, 66.28) (7.667, 65.8721) (7.5744, 65.6699) knots 0 0 0 0 0.067242 0.133324 0.133324 0.133324 0.133324
  spline S167 degree 3 poles (7.5744, 65.6699) (7.459, 65.4813) (7.2281, 65.1038) (6.8829, 64.8269) (6.7102, 64.6884) knots 0 0 0 0 0.065793 0.131657 0.131657 0.131657 0.131657
  spline S168 degree 3 poles (6.7102, 64.6884) (6.5517, 64.5887) (6.202, 64.3687) (5.8077, 64.244) (5.592, 64.1757) knots 0 0 0 0 0.055946 0.123455 0.123455 0.123455 0.123455
  spline S169 degree 3 poles (5.592, 64.1757) (5.3487, 64.1145) (4.8503, 63.9891) (4.3365, 63.9737) (4.0735, 63.9658) knots 0 0 0 0 0.075035 0.153702 0.153702 0.153702 0.153702
  spline S170 degree 3 poles (4.0735, 63.9658) (3.6883, 63.977) (2.9576, 63.9983) (2.2599, 64.2149) (1.9299, 64.3174) knots 0 0 0 0 0.11496 0.218119 0.218119 0.218119 0.218119
  spline S171 degree 3 poles (1.9299, 64.3174) (1.649, 64.4364) (1.1263, 64.6578) (0.7443, 65.076) (0.5676, 65.2695) knots 0 0 0 0 0.090247 0.167948 0.167948 0.167948 0.167948
  spline S172 degree 3 poles (0.5676, 65.2695) (0.4307, 65.4984) (0.1328, 65.9966) (0.022, 66.5674) (-0.0379, 66.8759) knots 0 0 0 0 0.079396 0.172838 0.172838 0.172838 0.172838
  line L120 (-0.0379, 66.8759) -> (1.6809, 67.1103)
  spline S173 degree 3 poles (1.6809, 67.1103) (1.7352, 66.8607) (1.8405, 66.3773) (2.1904, 66.0288) (2.3596, 65.8603) knots 0 0 0 0 0.074855 0.144953 0.144953 0.144953 0.144953
  spline S174 degree 3 poles (2.3596, 65.8603) (2.5799, 65.7296) (3.067, 65.4406) (3.6353, 65.4215) (3.9465, 65.4111) knots 0 0 0 0 0.075664 0.167297 0.167297 0.167297 0.167297
  spline S175 degree 3 poles (3.9465, 65.4111) (4.3003, 65.414) (4.9097, 65.4189) (5.4488, 65.6955) (5.675, 65.8115) knots 0 0 0 0 0.104241 0.179577 0.179577 0.179577 0.179577
  spline S176 degree 3 poles (5.675, 65.8115) (5.8258, 65.9449) (6.1111, 66.1972) (6.1665, 66.5723) (6.1926, 66.749) knots 0 0 0 0 0.05827 0.110201 0.110201 0.110201 0.110201
  spline S177 degree 3 poles (6.1926, 66.749) (6.1835, 66.8603) (6.1652, 67.0839) (6.0404, 67.2705) (5.9778, 67.3642) knots 0 0 0 0 0.032912 0.066134 0.066134 0.066134 0.066134
  spline S178 degree 3 poles (5.9778, 67.3642) (5.8903, 67.4568) (5.6987, 67.6593) (5.4429, 67.7719) (5.3039, 67.833) knots 0 0 0 0 0.037826 0.08282 0.08282 0.08282 0.08282
  spline S179 degree 3 poles (5.3039, 67.833) (5.1308, 67.8875) (4.6169, 68.0495) (4.0964, 68.1894) (3.7512, 68.2822) knots 0 0 0 0 0.054441 0.161656 0.161656 0.161656 0.161656
  spline S180 degree 3 poles (3.7512, 68.2822) (3.2203, 68.4232) (2.3405, 68.6568) (1.4871, 68.9725) (1.1487, 69.0976) knots 0 0 0 0 0.164675 0.27286 0.27286 0.27286 0.27286
  spline S181 degree 3 poles (1.1487, 69.0976) (0.9178, 69.213) (0.4663, 69.4388) (0.1473, 69.8295) (-0.0086, 70.0205) knots 0 0 0 0 0.076456 0.14952 0.14952 0.14952 0.14952
  spline S182 degree 3 poles (-0.0086, 70.0205) (-0.1309, 70.2417) (-0.3894, 70.7089) (-0.415, 71.2431) (-0.4285, 71.5244) knots 0 0 0 0 0.074822 0.158007 0.158007 0.158007 0.158007
  spline S183 degree 3 poles (-0.4285, 71.5244) (-0.4059, 71.815) (-0.3599, 72.4051) (-0.0653, 72.9189) (0.0842, 73.1797) knots 0 0 0 0 0.086284 0.175226 0.175226 0.175226 0.175226
  spline S184 degree 3 poles (0.0842, 73.1797) (0.2791, 73.426) (0.6826, 73.9358) (1.2635, 74.2292) (1.5637, 74.3808) knots 0 0 0 0 0.093067 0.192613 0.192613 0.192613 0.192613
  spline S185 degree 3 poles (1.5637, 74.3808) (1.9036, 74.5047) (2.6099, 74.762) (3.3614, 74.7907) (3.7512, 74.8056) knots 0 0 0 0 0.107841 0.22405 0.22405 0.22405 0.22405
  spline S186 degree 3 poles (3.7512, 74.8056) (4.3603, 74.7884) (5.46, 74.7574) (6.4089, 74.21) (6.8323, 73.9658) knots 0 0 0 0 0.179334 0.323794 0.323794 0.323794 0.323794
  spline S187 degree 3 poles (6.8323, 73.9658) (7.1559, 73.6374) (7.8437, 72.9395) (8.0667, 71.9824) (8.1848, 71.4756) knots 0 0 0 0 0.135648 0.28832 0.28832 0.28832 0.28832
  line L121 (11.9153, 62.2763) -> (11.9153, 60.2549)
  line L122 (11.9153, 60.2549) -> (10.1575, 60.2549)
  line L123 (10.1575, 60.2549) -> (10.1575, 62.2763)
  line L124 (10.1575, 62.2763) -> (11.9153, 62.2763)
  line L125 (29.7082, 78.5459) -> (29.7082, 64.2002)
  line L126 (29.7082, 64.2002) -> (28.1067, 64.2002)
  line L127 (28.1067, 64.2002) -> (28.1067, 65.5478)
  spline S188 degree 3 poles (28.1067, 65.5478) (27.9177, 65.304) (27.5563, 64.8377) (27.0628, 64.5152) (26.8274, 64.3613) knots 0 0 0 0 0.091799 0.17557 0.17557 0.17557 0.17557
  spline S189 degree 3 poles (26.8274, 64.3613) (26.5684, 64.246) (26.0189, 64.0015) (25.4171, 63.9781) (25.0989, 63.9658) knots 0 0 0 0 0.084252 0.178765 0.178765 0.178765 0.178765
  spline S190 degree 3 poles (25.0989, 63.9658) (24.673, 63.9917) (23.8395, 64.0425) (23.1113, 64.45) (22.7551, 64.6494) knots 0 0 0 0 0.126163 0.246958 0.246958 0.246958 0.246958
  spline S191 degree 3 poles (22.7551, 64.6494) (22.4352, 64.9057) (21.7786, 65.432) (21.4106, 66.1896) (21.2219, 66.5781) knots 0 0 0 0 0.121368 0.249146 0.249146 0.249146 0.249146
  spline S192 degree 3 poles (21.2219, 66.5781) (21.071, 67.0089) (20.7615, 67.8924) (20.7237, 68.8282) (20.7043, 69.3076) knots 0 0 0 0 0.136145 0.279187 0.279187 0.279187 0.279187
  spline S193 degree 3 poles (20.7043, 69.3076) (20.7248, 69.8173) (20.7643, 70.8033) (21.109, 71.7274) (21.2756, 72.1738) knots 0 0 0 0 0.151918 0.293913 0.293913 0.293913 0.293913
  spline S194 degree 3 poles (21.2756, 72.1738) (21.4833, 72.5711) (21.8896, 73.3481) (22.5923, 73.8712) (22.9358, 74.1269) knots 0 0 0 0 0.132578 0.259289 0.259289 0.259289 0.259289
  spline S195 degree 3 poles (22.9358, 74.1269) (23.2998, 74.3249) (24.0153, 74.7139) (24.827, 74.7754) (25.2258, 74.8056) knots 0 0 0 0 0.122747 0.241277 0.241277 0.241277 0.241277
  spline S196 degree 3 poles (25.2258, 74.8056) (25.5078, 74.792) (26.0568, 74.7653) (26.5588, 74.5428) (26.803, 74.4345) knots 0 0 0 0 0.083889 0.163269 0.163269 0.163269 0.163269
  spline S197 degree 3 poles (26.803, 74.4345) (27.0235, 74.305) (27.4546, 74.0517) (27.7877, 73.6791) (27.9504, 73.497) knots 0 0 0 0 0.076211 0.148977 0.148977 0.148977 0.148977
  line L128 (27.9504, 73.497) -> (27.9504, 78.5459)
  line L129 (27.9504, 78.5459) -> (29.7082, 78.5459)
  line L130 (9.8411, 53.1958) -> (8.4788, 53.3643)
  spline S198 degree 3 poles (8.4788, 53.3643) (8.6039, 53.7359) (8.8461, 54.4552) (9.4033, 54.969) (9.6726, 55.2173) knots 0 0 0 0 0.115551 0.223613 0.223613 0.223613 0.223613
  spline S199 degree 3 poles (9.6726, 55.2173) (9.9951, 55.4094) (10.6796, 55.8172) (11.4773, 55.8559) (11.8992, 55.8765) knots 0 0 0 0 0.110875 0.235384 0.235384 0.235384 0.235384
  spline S200 degree 3 poles (11.8992, 55.8765) (12.4301, 55.8413) (13.4453, 55.774) (14.2308, 55.1318) (14.6055, 54.8254) knots 0 0 0 0 0.155225 0.296837 0.296837 0.296837 0.296837
  spline S201 degree 3 poles (14.6055, 54.8254) (14.8966, 54.4193) (15.5257, 53.5417) (15.5774, 52.459) (15.6052, 51.8774) knots 0 0 0 0 0.146839 0.31723 0.31723 0.31723 0.31723
  spline S202 degree 3 poles (15.6052, 51.8774) (15.5778, 51.2766) (15.5269, 50.1613) (14.8888, 49.2506) (14.5945, 48.8306) knots 0 0 0 0 0.176138 0.326947 0.326947 0.326947 0.326947
  spline S203 degree 3 poles (14.5945, 48.8306) (14.2265, 48.5145) (13.4725, 47.8669) (12.4803, 47.7873) (11.9724, 47.7466) knots 0 0 0 0 0.141726 0.290335 0.290335 0.290335 0.290335
  spline S204 degree 3 poles (11.9724, 47.7466) (11.4798, 47.7871) (10.5143, 47.8664) (9.7821, 48.4989) (9.4236, 48.8086) knots 0 0 0 0 0.144189 0.28257 0.28257 0.28257 0.28257
  spline S205 degree 3 poles (9.4236, 48.8086) (9.1357, 49.2205) (8.511, 50.114) (8.4615, 51.2074) (8.4348, 51.7969) knots 0 0 0 0 0.147764 0.320562 0.320562 0.320562 0.320562
  spline S206 degree 3 poles (8.4348, 51.7969) (8.4353, 51.8457) (8.4364, 51.9629) (8.44, 52.0801) (8.4421, 52.1484) knots 0 0 0 0 0.01465 0.035165 0.035165 0.035165 0.035165
  line L131 (8.4421, 52.1484) -> (14.2429, 52.1484)
  spline S207 degree 3 poles (14.2429, 52.1484) (14.2048, 52.539) (14.1345, 53.2596) (13.7116, 53.8438) (13.5178, 54.1113) knots 0 0 0 0 0.115238 0.212619 0.212619 0.212619 0.212619
  spline S208 degree 3 poles (13.5178, 54.1113) (13.2856, 54.31) (12.8169, 54.711) (12.2021, 54.7652) (11.8919, 54.7925) knots 0 0 0 0 0.089299 0.180262 0.180262 0.180262 0.180262
  spline S209 degree 3 poles (11.8919, 54.7925) (11.6622, 54.7789) (11.218, 54.7526) (10.8377, 54.5227) (10.6541, 54.4116) knots 0 0 0 0 0.067871 0.131252 0.131252 0.131252 0.131252
  spline S210 degree 3 poles (10.6541, 54.4116) (10.4885, 54.2553) (10.1259, 53.913) (9.9413, 53.4483) (9.8411, 53.1958) knots 0 0 0 0 0.067501 0.147835 0.147835 0.147835 0.147835
  line L132 (44.3455, 55.7007) -> (44.3455, 47.9224)
  line L133 (44.3455, 47.9224) -> (43.1589, 47.9224)
  line L134 (43.1589, 47.9224) -> (43.1589, 49.1016)
  spline S211 degree 3 poles (43.1589, 49.1016) (43.0268, 48.862) (42.802, 48.4545) (42.4609, 48.1399) (42.3203, 48.0103) knots 0 0 0 0 0.081375 0.138409 0.138409 0.138409 0.138409
  spline S212 degree 3 poles (42.3203, 48.0103) (42.1892, 47.9333) (41.9276, 47.78) (41.6252, 47.7577) (41.4744, 47.7466) knots 0 0 0 0 0.044958 0.089666 0.089666 0.089666 0.089666
  spline S213 degree 3 poles (41.4744, 47.7466) (41.246, 47.7676) (40.7646, 47.812) (40.3417, 48.0476) (40.1194, 48.1714) knots 0 0 0 0 0.068034 0.143398 0.143398 0.143398 0.143398
  line L135 (40.1194, 48.1714) -> (40.5735, 49.3945)
  spline S214 degree 3 poles (40.5735, 49.3945) (40.7312, 49.3113) (41.0346, 49.151) (41.3762, 49.1226) (41.5403, 49.1089) knots 0 0 0 0 0.052874 0.101739 0.101739 0.101739 0.101739
  spline S215 degree 3 poles (41.5403, 49.1089) (41.6806, 49.1197) (41.9612, 49.1413) (42.1982, 49.2931) (42.3167, 49.3689) knots 0 0 0 0 0.041528 0.083017 0.083017 0.083017 0.083017
  spline S216 degree 3 poles (42.3167, 49.3689) (42.4239, 49.4662) (42.6451, 49.667) (42.7522, 49.9464) (42.8074, 50.0903) knots 0 0 0 0 0.042806 0.088343 0.088343 0.088343 0.088343
  spline S217 degree 3 poles (42.8074, 50.0903) (42.8715, 50.3344) (43.0038, 50.8385) (43.0192, 51.3596) (43.0271, 51.6284) knots 0 0 0 0 0.075431 0.155819 0.155819 0.155819 0.155819
  line L136 (43.0271, 51.6284) -> (43.0271, 55.7007)
  line L137 (43.0271, 55.7007) -> (44.3455, 55.7007)
  line L138 (53.9622, 54.5215) -> (53.7717, 55.686)
  spline S218 degree 3 poles (53.7717, 55.686) (53.947, 55.7202) (54.2761, 55.7843) (54.6112, 55.7972) (54.7678, 55.8032) knots 0 0 0 0 0.053462 0.100428 0.100428 0.100428 0.100428
  spline S219 degree 3 poles (54.7678, 55.8032) (54.9835, 55.7991) (55.3696, 55.7916) (55.7244, 55.6422) (55.8811, 55.5762) knots 0 0 0 0 0.063973 0.114534 0.114534 0.114534 0.114534
  spline S220 degree 3 poles (55.8811, 55.5762) (56.0022, 55.4967) (56.2367, 55.3428) (56.3722, 55.0977) (56.4378, 54.9792) knots 0 0 0 0 0.042726 0.08272 0.08272 0.08272 0.08272
  spline S221 degree 3 poles (56.4378, 54.9792) (56.4841, 54.7887) (56.608, 54.2786) (56.6024, 53.7524) (56.5989, 53.4228) knots 0 0 0 0 0.058662 0.156981 0.156981 0.156981 0.156981
  line L139 (56.5989, 53.4228) -> (56.5989, 48.9478)
  line L140 (56.5989, 48.9478) -> (57.5657, 48.9478)
  line L141 (57.5657, 48.9478) -> (57.5657, 47.9224)
  line L142 (57.5657, 47.9224) -> (56.5989, 47.9224)
  line L143 (56.5989, 47.9224) -> (56.5989, 45.9961)
  line L144 (56.5989, 45.9961) -> (55.2879, 45.2051)
  line L145 (55.2879, 45.2051) -> (55.2879, 47.9224)
  line L146 (55.2879, 47.9224) -> (53.9622, 47.9224)
  line L147 (53.9622, 47.9224) -> (53.9622, 48.9478)
  line L148 (53.9622, 48.9478) -> (55.2879, 48.9478)
  line L149 (55.2879, 48.9478) -> (55.2879, 53.4961)
  spline S222 degree 3 poles (55.2879, 53.4961) (55.2898, 53.6514) (55.2929, 53.8962) (55.2382, 54.1342) (55.2183, 54.2212) knots 0 0 0 0 0.046358 0.073057 0.073057 0.073057 0.073057
  spline S223 degree 3 poles (55.2183, 54.2212) (55.1911, 54.2723) (55.136, 54.376) (55.0399, 54.4434) (54.9912, 54.4775) knots 0 0 0 0 0.017119 0.034679 0.034679 0.034679 0.034679
  spline S224 degree 3 poles (54.9912, 54.4775) (54.9283, 54.5052) (54.7853, 54.5681) (54.6286, 54.5711) (54.5408, 54.5728) knots 0 0 0 0 0.020424 0.046442 0.046442 0.046442 0.046442
  spline S225 degree 3 poles (54.5408, 54.5728) (54.4558, 54.5697) (54.2621, 54.5629) (54.07, 54.5364) (53.9622, 54.5215) knots 0 0 0 0 0.025484 0.058121 0.058121 0.058121 0.058121
  line L150 (74.99, 55.7007) -> (74.99, 44.9634)
  line L151 (74.99, 44.9634) -> (67.2263, 44.9634)
  line L152 (67.2263, 44.9634) -> (67.2263, 46.2305)
  line L153 (67.2263, 46.2305) -> (73.5691, 46.2305)
  line L154 (73.5691, 46.2305) -> (73.5691, 49.519)
  line L155 (73.5691, 49.519) -> (67.6292, 49.519)
  line L156 (67.6292, 49.519) -> (67.6292, 50.7788)
  line L157 (67.6292, 50.7788) -> (73.5691, 50.7788)
  line L158 (73.5691, 50.7788) -> (73.5691, 54.4336)
  line L159 (73.5691, 54.4336) -> (66.9773, 54.4336)
  line L160 (66.9773, 54.4336) -> (66.9773, 55.7007)
  line L161 (66.9773, 55.7007) -> (74.99, 55.7007)
  line L162 (68.807, 40.8932) -> (68.807, 35.7077)
  line L163 (68.807, 35.7077) -> (68.016, 35.7077)
  line L164 (68.016, 35.7077) -> (68.016, 36.445)
  spline S226 degree 3 poles (68.016, 36.445) (67.8018, 36.1958) (67.3672, 35.69) (66.7027, 35.624) (66.3656, 35.5905) knots 0 0 0 0 0.094776 0.192358 0.192358 0.192358 0.192358
  spline S227 degree 3 poles (66.3656, 35.5905) (66.2141, 35.5968) (65.9182, 35.6092) (65.6397, 35.7098) (65.5038, 35.759) knots 0 0 0 0 0.04518 0.088272 0.088272 0.088272 0.088272
  spline S228 degree 3 poles (65.5038, 35.759) (65.3834, 35.8162) (65.157, 35.924) (64.9925, 36.1126) (64.9154, 36.2009) knots 0 0 0 0 0.039495 0.074282 0.074282 0.074282 0.074282